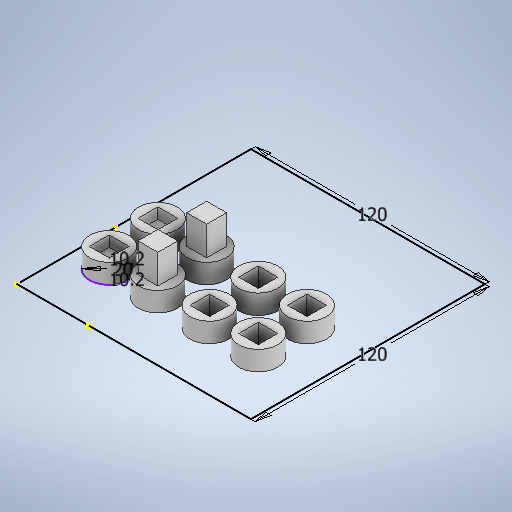
# Autodesk Inventor part: print1030_1
Saved by Autodesk Inventor 2025.1 (Build 291241000, 241)
## iProperties
Created: 2024-10-30
Part Number: print1030_1
Material: 一般
Document SubType Name: Modeling
Designer: youtian
Density: 1 g/cm^3
Appearance: 預設
Author: youtian
Autodesk Inventor part; units mm, degrees
ref_plane "YZ Plane" through (0, 0, 0) normal (1, 0, 0) x (0, 1, 0)
ref_plane "XZ Plane" through (0, 0, 0) normal (0, 1, 0) x (-1, 0, 0)
ref_plane "XY Plane" through (0, 0, 0) normal (0, 0, 1) x (1, 0, 0)
sketch "草圖1" plane through (0, 0, 0) normal (0, 1, 0) x (-1, 0, 0)
  line L0 (0, 0) -> (-120, 0)
  line L1 (-120, 0) -> (-120, -120)
  line L2 (-120, -120) -> (0, -120)
  line L3 (0, -120) -> (0, 0)
  dimension "d0" = 120
  dimension "d1" = 120
  constraints: 8 end point, 2 parallel, 1 horizontal, 1 perpendicular
  measures "d0" distance of L2.end L1.end
  measures "d1" distance of L1.end L0.end
sketch "草圖2" plane through (0, 0, 0) normal (0, 1, 0) x (-1, 0, 0)
  line L0 (-11.7915, -25.267) -> (-21.9915, -25.267)
  line L1 (-21.9915, -25.267) -> (-21.9915, -35.467)
  line L2 (-21.9915, -35.467) -> (-11.7915, -35.467)
  line L3 (-11.7915, -35.467) -> (-11.7915, -25.267)
  circle A0 centre (-16.8915, -30.367) radius 10
  point P0 (0, 0)
  dimension "d11" = 10.2
  dimension "d12" = 10.2
  dimension "d13" = 20
  constraints: 8 end point, 2 parallel, 1 centre point, 1 horizontal, 1 perpendicular
  measures "d11" distance of L2.end L1.end
  measures "d12" distance of L1.end L0.end
  measures "d13" diameter of A0
extrude "擠出1" add sketch "草圖2" along normal blind 10
extrude "擠出2" add sketch "草圖2" along normal blind 4.5 contours L3 L2 L1 L0
pattern_linear "矩形陣列1" count 2 spacing 25 along (0, 0, -1) count 2 spacing 25 along (1, 0, 0) of "擠出1", "擠出2"
sketch "草圖3" plane through (0, 0, 0) normal (0, 1, 0) x (-1, 0, 0)
  circle A0 centre (-68.8014, -29.9583) radius 10
  line L0 (-63.8014, -24.9583) -> (-73.8014, -24.9583)
  line L1 (-73.8014, -24.9583) -> (-73.8014, -34.9583)
  line L2 (-73.8014, -34.9583) -> (-63.8014, -34.9583)
  line L3 (-63.8014, -34.9583) -> (-63.8014, -24.9583)
  line L4 (-63.8014, -24.9583) -> (-73.8014, -34.9583) construction
  line L5 (-73.8014, -24.9583) -> (-63.8014, -34.9583) construction
  point P0 (0, 0)
  dimension "d32" = 20
  dimension "d33" = 10
  dimension "d34" = 10
  constraints: 12 end point, 2 midpoint, 2 parallel, 1 centre point, 1 horizontal, 1 perpendicular
  measures "d32" diameter of A0
  measures "d33" distance of L2.end L1.end
  measures "d34" distance of L1.end L0.end
extrude "擠出3" add sketch "草圖3" along normal blind 10
pattern_linear "矩形陣列2" count 2 spacing 25 along (0, 0, -1) count 2 spacing 25 along (1, 0, 0) of "擠出3"
sketch "草圖4" plane through (36.7915, 4.5, -60.467) normal (0, 1, 0) x (1, 0, 0)
  line L0 (0, -10.2) -> (0, 0) projected
  line L1 (10.2, 0) -> (10.2, -10.2) projected
  line L2 (0, 0) -> (10.2, 0)
  line L3 (10.2, 0) -> (10.2, -10.2)
  line L4 (10.2, -10.2) -> (0, -10.2)
  line L5 (0, -10.2) -> (0, 0)
  point P0 (-36.7915, -60.467)
  constraints: 8 end point, 2 parallel, 1 horizontal, 1 perpendicular
extrude "擠出4" add sketch "草圖4" along normal blind 20.5
sketch "草圖5" plane through (36.7915, 10, -50.267) normal (0, 0, 1) x (1, 0, 0)
  point P0 (-36.7915, -10)
sketch "草圖6" plane through (36.7915, 4.5, -35.467) normal (1, 0, 0) x (0, 0, -1)
  point P0 (-35.467, -4.5)
pattern_linear "矩形陣列3" count 2 spacing 25 along (0, 0, 1) of "擠出4"
